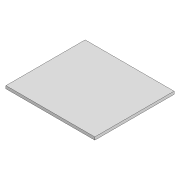
# Autodesk Inventor part: TB_Sides
Saved by Autodesk Inventor 2021.3 (Build 253353000, 353)
## iProperties
Created: 2021-11-26
Part Number: TB_Sides
Material: Generic
Document SubType Name: Modeling
Designer: wbrooks
Density: 1 g/cm^3
Appearance: Default
Author: wbrooks
Autodesk Inventor part; units mm, degrees
ref_plane "YZ Plane" through (0, 0, 0) normal (1, 0, 0) x (0, 1, 0)
ref_plane "XZ Plane" through (0, 0, 0) normal (0, 1, 0) x (-1, 0, 0)
ref_plane "XY Plane" through (0, 0, 0) normal (0, 0, 1) x (1, 0, 0)
sketch "Sketch1" plane through (0, 0, 0) normal (0, 1, 0) x (-1, 0, 0)
  line L0 (-189.7063, 169.0687) -> (189.7062, 169.0687)
  line L1 (189.7062, 169.0687) -> (189.7062, -169.0688)
  line L2 (189.7062, -169.0688) -> (-189.7062, -169.0688)
  line L3 (-189.7062, -169.0688) -> (-189.7063, 169.0687)
  line L4 (-189.7063, 169.0687) -> (189.7062, -169.0688) construction
  line L5 (189.7062, 169.0687) -> (-189.7062, -169.0688) construction
  point P0 (0, 0)
  dimension "d2" = 338.1375
  dimension "d3" = 379.4125
  constraints: 12 end point, 2 midpoint, 2 parallel, 1 horizontal, 1 perpendicular
  measures "d2" distance of L0.end L1.end
  measures "d3" distance of L0.start L0.end
extrude "Extrusion1" add sketch "Sketch1" along normal mid plane 11.9062
body "Solid1"
